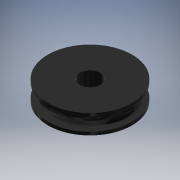
# Autodesk Inventor part: 0.5OD_Pulley
Saved by Autodesk Inventor 2019 (Build 230136000, 136)
## iProperties
Created: 2021-02-23
Part Number: 0.5OD_Pulley
Material: ABS Plastic
Document SubType Name: Modeling
Designer: zhanb
Density: 1.06 g/cm^3
Appearance: Smooth - Black
Author: zhanb
Autodesk Inventor part; units mm, degrees
ref_plane "YZ Plane" through (0, 0, 0) normal (1, 0, 0) x (0, 1, 0)
ref_plane "XZ Plane" through (0, 0, 0) normal (0, 1, 0) x (-1, 0, 0)
ref_plane "XY Plane" through (0, 0, 0) normal (0, 0, 1) x (1, 0, 0)
sketch "Sketch1" plane through (0, 0, 0) normal (1, 0, 0) x (0, 1, 0)
  line L0 (-2.3813, 10.3315) -> (-2.3813, 0) construction
  line L1 (-2.3813, 0) -> (0, 0) construction
  line L2 (2.3813, 0) -> (2.3812, 10.3315)
  line L3 (2.3812, 10.3315) -> (0, 10.3315)
  line L4 (-2.3813, 10.3315) -> (2.3813, 0) construction
  line L5 (-2.3813, 0) -> (2.3812, 10.3315) construction
  line L6 (0, 9.525) -> (0, 7.9121)
  line L7 (0, 7.9121) -> (0, 10.3315)
  line L8 (0, 10.3315) -> (-2.3813, 10.3315) construction
  line L9 (0, 0) -> (2.3813, 0)
  line L10 (0, 7.9121) -> (0, 0)
  arc A0 (0, 7.9121) -> (1.6129, 9.525) centre (0, 9.525) ccw
  line L11 (1.6129, 9.525) -> (1.6129, 10.3315)
  point P0 (0, 5.1657)
  point P1 (0, 5.1657)
  dimension "d2" = 1.6129
  dimension "d4" = 2.3813
  dimension "d5" = 0.8065
  dimension "d10" = 9.525
  constraints: 24 end point, 5 parallel, 4 vertical, 3 midpoint, 3 point on line, 2 perpendicular, 2 point on circle, 1 centre point, 1 tangent
  measures "d2" radius of A0
  measures "d4" distance of L2.end L3.end
  measures "d5" distance of L3.end L6.start
  measures "d10" distance from line of L9 L6.start
revolve "Revolution1" add sketch "Sketch1" angle 360 about axis through (0, 0, 0) along (0, 1, 0) contours L9 L10 A0 L11 L3 L2
mirror "Mirror1" about plane through (0, 0, 7.9121) normal (0, -1, 0) of "Revolution1"
sketch "Sketch2" plane through (0, -2.3813, 0) normal (0, -1, 0) x (1, 0, 0)
  circle A0 centre (0, 0) radius 2.54
  point P0 (0, 0)
  dimension "d7" = 5.08
  constraints: 1 centre point, 1 coincident
  measures "d7" diameter of A0
extrude "Extrusion1" cut sketch "Sketch2" against normal through all
equation "\"d5\" = 0.5 * d2"
body "Solid1"
